Autodesk Inventor part; units mm, degrees
note: some values were not read from the file. Chosen so that the rebuilt part matches the saved one: direction of "Hole2".
(part 8 of 18)
  ellipse E33 centre (-86.9882, -23.0551) end of major axis (-85.4887, -23.0929) minor radius 0.2511 (-85.5525, -23.1627) -> (-87.7819, -22.8225) ccw
  ellipse E34 centre (-87.3359, -36.8531) end of major axis (-88.1356, -36.833) minor radius 0.1339 (-87.4465, -36.7177) -> (-87.4665, -36.7178) ccw
  ellipse E35 centre (-87.3607, -37.8387) end of major axis (-87.8606, -37.8261) minor radius 0.0837 (-87.1122, -37.9174) -> (-87.0891, -37.9156) ccw
  ellipse E36 centre (-87.3607, -37.8387) end of major axis (-86.8609, -37.8513) minor radius 0.0837 (-87.0358, -37.783) -> (-87.287, -37.7577) ccw
  line L78 (-105.3004, -36.9196) -> (-105.1861, -36.9462)
  ellipse E37 centre (-105.7695, -36.9513) end of major axis (-106.5469, -36.7626) minor radius 0.1369 (-105.4577, -36.8957) -> (-105.4762, -36.8899) ccw
  ellipse E38 centre (-106.002, -37.9088) end of major axis (-105.5161, -38.0267) minor radius 0.0856 (-105.735, -38.0451) -> (-105.8816, -37.8518) ccw
  ellipse E39 centre (-103.1271, -36.0379) end of major axis (-103.8852, -35.7824) minor radius 0.0023 (-103.715, -35.8383) -> (-103.8852, -35.7824) ccw
  line L79 (-101.9076, -36.989) -> (-102.0626, -37.449)
  line L80 (-103.888, -35.7905) -> (-103.8852, -35.7824)
  line L81 (-101.0026, -34.3039) -> (-99.7688, -30.6433)
  line L82 (-101.8233, -37.3232) -> (-102.0626, -37.449)
  line L83 (-102.0626, -37.449) -> (-102.0859, -37.4413)
  line L84 (-102.3857, -37.3402) -> (-102.0626, -37.449)
  line L85 (-90.6472, -35.9583) -> (-90.4914, -35.9237)
  ellipse E40 centre (-90.4117, -35.9087) end of major axis (-89.6305, -35.736) minor radius 0.0026 (-90.363, -35.8954) -> (-90.4914, -35.9237) ccw
  ellipse E41 centre (-90.4117, -35.9087) end of major axis (-89.6305, -35.736) minor radius 0.0026 (-90.2467, -35.8697) -> (-90.36, -35.8947) ccw
  ellipse E42 centre (-90.4117, -35.9087) end of major axis (-89.6305, -35.736) minor radius 0.0026 (-89.6305, -35.736) -> (-90.0478, -35.8259) ccw
  line L86 (-89.6301, -35.738) -> (-89.6305, -35.736)
  ellipse E43 centre (-87.6822, -37.9556) end of major axis (-86.8871, -37.8673) minor radius 0.2631 (-88.3686, -38.1574) -> (-88.2224, -38.2033) ccw
  ellipse E44 centre (-87.6822, -37.9556) end of major axis (-86.8871, -37.8673) minor radius 0.2631 (-87.1208, -38.0875) -> (-86.9563, -37.9921) ccw
  ellipse E45 centre (-106.3209, -37.9556) end of major axis (-107.116, -37.8673) minor radius 0.2631 (-106.8502, -37.7057) -> (-107.0012, -37.7511) ccw
  ellipse E46 centre (-106.3209, -37.9556) end of major axis (-107.116, -37.8673) minor radius 0.2631 (-107.0315, -37.7663) -> (-107.0404, -37.7715) ccw
  ellipse E47 centre (-106.3209, -37.9556) end of major axis (-107.116, -37.8673) minor radius 0.2631 (-107.107, -37.9186) -> (-106.8822, -38.0875) ccw
  ellipse E48 centre (-106.3209, -37.9556) end of major axis (-105.5258, -38.044) minor radius 0.2631 (-105.7807, -38.2033) -> (-105.6345, -38.1574) ccw
  line L87 (-92.5959, -36.6984) -> (-92.477, -36.6522)
  ellipse E49 centre (-91.0664, -36.1069) end of major axis (-90.3205, -35.8175) minor radius 0.0025 (-90.9446, -36.0571) -> (-90.9611, -36.0635) ccw
  ellipse E50 centre (-91.0664, -36.1069) end of major axis (-90.3205, -35.8175) minor radius 0.0025 (-90.8503, -36.0205) -> (-90.8987, -36.0393) ccw
  ellipse E51 centre (-91.0664, -36.1069) end of major axis (-90.3205, -35.8175) minor radius 0.0025 (-90.3205, -35.8175) -> (-90.3921, -35.8441) ccw
  line L88 (-92.2341, -37.6306) -> (-92.5959, -36.6984)
  ellipse E52 centre (-90.3428, -37.9714) end of major axis (-91.0886, -38.2609) minor radius 0.0025 (-90.6436, -38.0858) -> (-90.6333, -38.0866) ccw
  line L89 (-91.0886, -38.2609) -> (-91.4504, -37.3286)
  line L90 (-90.3147, -35.8327) -> (-90.3205, -35.8175)
  line L91 (-92.5959, -36.6984) -> (-94.5282, -31.7193)
  line L92 (-91.4495, -37.3309) -> (-92.2341, -37.6306)
  line L93 (-92.2341, -37.6306) -> (-92.5845, -37.4453)
  ellipse E53 centre (-92.2567, -37.3201) end of major axis (-93.1315, -36.9354) minor radius 0.2554 (-93.1284, -37.0086) -> (-92.5845, -37.4453) ccw
  line L94 (-93.1284, -37.0086) -> (-94.6292, -33.1414)
  ellipse E54 centre (-90.7046, -37.0392) end of major axis (-91.4504, -37.3286) minor radius 0.0025 (-91.304, -37.2702) -> (-91.4504, -37.3286) ccw
  line L95 (-92.2341, -37.6306) -> (-91.3087, -37.2712)
  ellipse E55 centre (-90.3428, -37.9714) end of major axis (-90.8089, -38.1523) minor radius 0.0015 (-90.6412, -38.086) -> (-90.6357, -38.0864) ccw
  ellipse E56 centre (-88.3729, -36.9958) end of major axis (-89.1416, -37.2174) minor radius 0.1461 (-88.5826, -36.9079) -> (-88.8145, -36.9941) ccw
  line L96 (-88.8154, -36.977) -> (-88.5903, -36.9086)
  ellipse E57 centre (-88.1005, -37.9405) end of major axis (-88.5809, -38.079) minor radius 0.0913 (-88.1238, -37.8521) -> (-88.2596, -38.0743) ccw
  ellipse E58 centre (-88.1005, -37.9405) end of major axis (-88.8692, -38.1621) minor radius 0.1461 (-88.4277, -37.8939) -> (-88.3686, -38.1574) ccw
  line L97 (-88.8692, -38.1621) -> (-88.9803, -37.7768)
  line L98 (-96.3959, -34.9516) -> (-96.4243, -34.4948)
  line L99 (-101.4811, -37.3766) -> (-101.4038, -37.5126)
  line L100 (-101.4038, -37.5126) -> (-100.927, -37.4058)
  ellipse E59 centre (-99.6492, -37.9242) end of major axis (-100.4225, -38.1293) minor radius 0.1421 (-100.4225, -38.1293) -> (-100.0049, -38.1458) ccw
  line L101 (-100.4225, -38.1293) -> (-100.5976, -37.4691)
  line L102 (-106.2018, -35.7078) -> (-106.2106, -35.5345)
  line L103 (-105.4545, -35.6102) -> (-105.4515, -35.6707)
  ellipse E60 centre (-106.8036, -35.8807) end of major axis (-107.6025, -35.9211) minor radius 0.143 (-107.0863, -35.7606) -> (-107.6025, -35.9211) ccw
  line L104 (-106.806, -35.7377) -> (-105.2331, -35.6598)
  line L105 (-105.2331, -35.6598) -> (-105.2316, -35.6894)
  ellipse E61 centre (-106.7042, -37.846) end of major axis (-107.5032, -37.8864) minor radius 0.143 (-107.024, -37.7305) -> (-107.0468, -37.9921) ccw
  ellipse E62 centre (-106.7042, -37.846) end of major axis (-107.5032, -37.8864) minor radius 0.143 (-106.4334, -37.6981) -> (-106.7066, -37.703) ccw
  line L106 (-107.5032, -37.8864) -> (-107.6025, -35.9211)
  line L107 (-105.2331, -35.6598) -> (-105.2348, -35.6248)
  line L108 (-105.2865, -34.6021) -> (-105.328, -33.7811)
  line L109 (-106.4202, -35.7186) -> (-106.4309, -35.508)
  ellipse E63 centre (-107.4941, -22.222) end of major axis (-109.5814, -22.3275) minor radius 0.3735 (-108.146, -21.8986) -> (-109.5814, -22.3275) ccw
  ellipse E64 centre (-107.4494, -23.1063) end of major axis (-109.5367, -23.2119) minor radius 0.3735 (-108.1131, -22.7842) -> (-109.0841, -23.4189) ccw
  line L110 (-109.5814, -22.3275) -> (-109.5367, -23.2119)
  ellipse E65 centre (-107.4494, -23.1063) end of major axis (-108.9475, -23.1821) minor radius 0.2681 (-106.2292, -22.8909) -> (-108.7917, -23.2912) ccw
  ellipse E66 centre (-106.7042, -37.846) end of major axis (-107.2036, -37.8712) minor radius 0.0894 (-106.7198, -37.7573) -> (-106.8898, -37.9381) ccw
  line L111 (-103.5666, -35.7887) -> (-103.544, -35.3586)
  line L112 (-102.9282, -34.2217) -> (-102.9384, -34.416)
  line L113 (-102.9917, -35.4294) -> (-103.0151, -35.8748)
  ellipse E67 centre (-104.3252, -35.809) end of major axis (-105.1241, -35.767) minor radius 0.0026 (-104.4162, -35.8017) -> (-105.1241, -35.767) ccw
  line L114 (-104.4162, -35.8017) -> (-102.8537, -35.8832)
  line L115 (-102.8537, -35.8832) -> (-102.8551, -35.9105)
  ellipse E68 centre (-104.4302, -37.8062) end of major axis (-105.2291, -37.7643) minor radius 0.0026 (-104.7673, -37.7862) -> (-104.7579, -37.7914) ccw
  line L116 (-105.2291, -37.7643) -> (-105.1241, -35.767)
  line L117 (-102.8537, -35.8832) -> (-102.7674, -34.2418)
  line L118 (-103.7279, -35.7784) -> (-103.7155, -35.5431)
  ellipse E69 centre (-104.4302, -37.8062) end of major axis (-104.9295, -37.78) minor radius 0.0016 (-104.7651, -37.7874) -> (-104.7602, -37.7901) ccw
  line L119 (-91.8056, -35.8014) -> (-92.3575, -33.1978)
  ellipse E70 centre (-90.3624, -35.9507) end of major axis (-88.9928, -35.6604) minor radius 0.2113 (-90.91, -35.8661) -> (-90.9339, -35.8727) ccw
  line L120 (-90.9872, -35.5021) -> (-90.91, -35.8661)
  line L121 (-91.9378, -36.3888) -> (-91.8413, -36.3397)
  line L122 (-90.91, -35.8661) -> (-90.8335, -35.8271)
  line L123 (-91.9378, -36.3888) -> (-90.398, -36.0813)
  ellipse E71 centre (-90.3624, -35.9507) end of major axis (-89.5798, -35.7848) minor radius 0.1207 (-90.398, -36.0813) -> (-89.7408, -35.747) ccw
  line L124 (-89.7408, -35.747) -> (-90.657, -35.7482)
  line L125 (-91.7329, -37.3559) -> (-91.9378, -36.3888)
  ellipse E72 centre (-89.9524, -37.8848) end of major axis (-90.7351, -38.0507) minor radius 0.1207 (-90.6436, -38.0858) -> (-89.2358, -37.7862) ccw
  line L126 (-89.5781, -35.7926) -> (-89.5798, -35.7848)
  line L127 (-91.9378, -36.3888) -> (-92.609, -33.2223)
  line L128 (-91.7329, -37.3559) -> (-92.0546, -37.0982)
  ellipse E73 centre (-91.7375, -36.9369) end of major axis (-92.5311, -36.3716) minor radius 0.32 (-92.5473, -36.4923) -> (-92.0546, -37.0982) ccw
  line L129 (-92.5473, -36.4923) -> (-93.8742, -30.2315)
  line L130 (-91.7329, -37.3559) -> (-90.193, -37.0483)
  line L131 (-89.3251, -35.7753) -> (-89.3885, -35.2136)
  line L132 (-88.4512, -35.6057) -> (-88.4408, -35.6984)
  line L133 (-88.8708, -35.9234) -> (-88.0017, -35.8236)
  ellipse E74 centre (-87.9255, -35.8321) end of major axis (-87.1305, -35.7424) minor radius 0.017 (-87.1432, -35.7409) -> (-88.0017, -35.8236) ccw
  ellipse E75 centre (-87.7014, -37.819) end of major axis (-88.4963, -37.9087) minor radius 0.017 (-86.9791, -37.7305) -> (-88.4277, -37.8939) ccw
  line L134 (-89.5896, -35.7345) -> (-89.6468, -35.2274)
  ellipse E76 centre (-89.4829, -22.0228) end of major axis (-87.406, -21.7886) minor radius 0.0445 (-87.4742, -21.785) -> (-87.8996, -21.8153) ccw
  ellipse E77 centre (-89.382, -22.9169) end of major axis (-87.3052, -22.6827) minor radius 0.0445 (-87.376, -22.6792) -> (-87.7951, -22.7091) ccw
  ellipse E78 centre (-87.8134, -36.8256) end of major axis (-88.6084, -36.9152) minor radius 0.017 (-87.8896, -36.8171) -> (-88.5826, -36.9079) ccw
  line L135 (-88.8182, -36.9237) -> (-87.8896, -36.8171)
  ellipse E79 centre (-87.7014, -37.819) end of major axis (-88.1982, -37.8751) minor radius 0.0106 (-87.2268, -37.7624) -> (-88.1906, -37.8723) ccw
  line L136 (-95.4221, -34.9516) -> (-95.3724, -34.4948)
  line L137 (-93.3346, -36.8473) -> (-94.4853, -36.841)
  line L138 (-94.3267, -37.4213) -> (-93.0147, -37.4285)
  line L139 (-93.0147, -37.4285) -> (-92.9086, -37.2552)
  ellipse E80 centre (-93.5822, -37.2515) end of major axis (-92.8706, -37.0672) minor radius 0.3717 (-93.1865, -36.8589) -> (-93.3346, -36.8473) ccw
  ellipse E81 centre (-93.5822, -37.2515) end of major axis (-92.8706, -37.0672) minor radius 0.3717 (-92.9086, -37.2552) -> (-92.9039, -37.2474) ccw
  ellipse E82 centre (-94.7288, -37.9666) end of major axis (-93.9335, -38.0531) minor radius 0.2736 (-94.1139, -38.2002) -> (-93.9982, -38.1458) ccw
  line L140 (-98.4172, -34.9516) -> (-98.4669, -34.4948)
  ellipse E83 centre (-100.2771, -37.2761) end of major axis (-99.5693, -37.3693) minor radius 0.4004 (-100.4443, -36.8697) -> (-100.9668, -37.3091) ccw
  line L141 (-100.9854, -37.2376) -> (-101.0007, -37.0971)
  line L142 (-99.5135, -36.8252) -> (-100.4443, -36.8697)
  line L143 (-100.9668, -37.3091) -> (-100.8951, -37.4833)
  line L144 (-100.8951, -37.4833) -> (-99.6774, -37.4251)
  ellipse E84 centre (-99.2743, -37.9666) end of major axis (-100.0696, -38.0531) minor radius 0.2736 (-100.0049, -38.1458) -> (-99.8891, -38.2002) ccw
  ellipse E85 centre (-106.0776, -35.8321) end of major axis (-106.8726, -35.7424) minor radius 0.017 (-106.0833, -35.8143) -> (-106.8599, -35.7409) ccw
  line L145 (-106.0833, -35.8143) -> (-105.1322, -35.9214)
  ellipse E86 centre (-106.3017, -37.819) end of major axis (-107.0967, -37.7294) minor radius 0.017 (-105.5754, -37.8939) -> (-107.024, -37.7305) ccw
  line L146 (-104.4898, -35.7366) -> (-104.4319, -35.2234)
  ellipse E87 centre (-104.5202, -22.0228) end of major axis (-106.5971, -21.7886) minor radius 0.0445 (-106.1035, -21.8153) -> (-106.5971, -21.7886) ccw
  ellipse E88 centre (-104.6211, -22.9169) end of major axis (-106.6979, -22.6827) minor radius 0.0445 (-106.208, -22.7091) -> (-106.627, -22.6792) ccw
  line L147 (-106.1954, -36.8078) -> (-105.1848, -36.9215)
  ellipse E89 centre (-106.1897, -36.8256) end of major axis (-105.3947, -36.9152) minor radius 0.017 (-105.4205, -36.9079) -> (-106.1954, -36.8078) ccw
  ellipse E90 centre (-106.3017, -37.819) end of major axis (-106.7986, -37.763) minor radius 0.0106 (-105.8581, -37.8739) -> (-106.7505, -37.773) ccw
  line L148 (-103.1826, -35.8132) -> (-104.1672, -35.7504)
  ellipse E91 centre (-103.6407, -35.9507) end of major axis (-104.4233, -35.7848) minor radius 0.1207 (-104.1672, -35.7504) -> (-103.7453, -36.0513) ccw
  line L149 (-103.7453, -36.0513) -> (-102.2177, -36.3998)
  line L150 (-102.2177, -36.3998) -> (-102.4227, -37.3668)
  ellipse E92 centre (-104.0506, -37.8848) end of major axis (-104.8333, -37.7189) minor radius 0.1207 (-104.7673, -37.7862) -> (-103.3595, -38.0858) ccw
  line L151 (-104.425, -35.7926) -> (-104.4233, -35.7848)
  line L152 (-102.2505, -36.3764) -> (-102.2177, -36.3998)
  line L153 (-102.2177, -36.3998) -> (-101.5416, -33.2099)
  ellipse E93 centre (-102.2845, -36.9758) end of major axis (-101.4721, -36.4169) minor radius 0.2359 (-102.0808, -37.121) -> (-101.4724, -36.5094) ccw
  line L154 (-101.4046, -36.2006) -> (-100.1521, -30.2914)
  line L155 (-102.0808, -37.121) -> (-102.4227, -37.3668)
  line L156 (-103.9503, -37.0183) -> (-102.4227, -37.3668)
  line L157 (-91.0541, -35.879) -> (-91.0769, -35.4447)
  line L158 (-90.2308, -35.4655) -> (-90.216, -35.7476)
  line L159 (-91.2994, -35.892) -> (-89.73, -35.8092)
  ellipse E94 centre (-89.6779, -35.809) end of major axis (-88.879, -35.767) minor radius 0.0026 (-88.879, -35.767) -> (-89.73, -35.8092) ccw
  line L160 (-91.2968, -35.9413) -> (-91.2994, -35.892)
  ellipse E95 centre (-89.5729, -37.8062) end of major axis (-88.774, -37.7643) minor radius 0.0026 (-89.2452, -37.7914) -> (-89.2358, -37.7862) ccw
  line L161 (-88.774, -37.7643) -> (-88.879, -35.767)
  line L162 (-89.9702, -35.7439) -> (-89.9858, -35.4481)
  line L163 (-91.2994, -35.892) -> (-91.3855, -34.2529)
  ellipse E96 centre (-89.5729, -37.8062) end of major axis (-89.0736, -37.78) minor radius 0.0016 (-89.2428, -37.7901) -> (-89.238, -37.7874) ccw
  line L164 (-88.5794, -35.6942) -> (-88.5755, -35.6163)
  line L165 (-87.6584, -35.5185) -> (-87.6687, -35.7223)
  line L166 (-88.8445, -35.686) -> (-87.2794, -35.7344)
  ellipse E97 centre (-87.1995, -35.8807) end of major axis (-86.4005, -35.9211) minor radius 0.143 (-86.4005, -35.9211) -> (-86.9168, -35.7606) ccw
  line L167 (-88.8467, -35.7306) -> (-88.8445, -35.686)
  ellipse E98 centre (-87.2989, -37.846) end of major axis (-86.4999, -37.8864) minor radius 0.143 (-86.639, -37.959) -> (-86.9791, -37.7305) ccw
  line L168 (-86.4999, -37.8864) -> (-86.4005, -35.9211)
  line L169 (-87.4036, -35.7305) -> (-87.3912, -35.485)
  line L170 (-88.8445, -35.686) -> (-88.8346, -35.4897)
  line L171 (-88.7547, -33.9096) -> (-88.742, -33.6588)
  ellipse E99 centre (-86.509, -22.222) end of major axis (-84.4216, -22.3275) minor radius 0.3735 (-84.4216, -22.3275) -> (-85.857, -21.8986) ccw
  ellipse E100 centre (-86.5537, -23.1063) end of major axis (-84.4663, -23.2119) minor radius 0.3735 (-84.8558, -23.407) -> (-85.89, -22.7842) ccw
  line L172 (-84.4216, -22.3275) -> (-84.4663, -23.2119)
  ellipse E101 centre (-86.5537, -23.1063) end of major axis (-85.0556, -23.1821) minor radius 0.2681 (-85.1981, -23.287) -> (-87.7739, -22.8909) ccw
  ellipse E102 centre (-87.2989, -37.846) end of major axis (-86.7995, -37.8712) minor radius 0.0894 (-87.1133, -37.9381) -> (-87.2833, -37.7573) ccw
  line L173 (-92.9989, -37.4027) -> (-92.5139, -37.5)
  line L174 (-92.5139, -37.5) -> (-92.5046, -37.4875)
  ellipse E103 centre (-94.3538, -37.9242) end of major axis (-93.5806, -38.1293) minor radius 0.1421 (-93.9982, -38.1458) -> (-93.5806, -38.1293) ccw
  line L175 (-93.5806, -38.1293) -> (-93.3941, -37.4264)
  line L176 (-97.4502, -34.9516) -> (-97.4218, -34.4948)
  line L177 (-105.396, -36.9102) -> (-105.1873, -36.9692)
  ellipse E104 centre (-105.6302, -36.9958) end of major axis (-106.3989, -36.7741) minor radius 0.1461 (-105.1886, -36.9941) -> (-105.4205, -36.9079) ccw
  ellipse E105 centre (-105.9026, -37.9405) end of major axis (-105.4222, -38.079) minor radius 0.0913 (-105.7434, -38.0743) -> (-105.8793, -37.8521) ccw
  ellipse E106 centre (-105.9026, -37.9405) end of major axis (-105.1339, -38.1621) minor radius 0.1461 (-105.6345, -38.1574) -> (-105.5754, -37.8939) ccw
  line L178 (-105.1339, -38.1621) -> (-105.0228, -37.7768)
  ellipse E107 centre (-102.9367, -36.1069) end of major axis (-103.6825, -35.8175) minor radius 0.0025 (-103.6284, -35.8375) -> (-103.6825, -35.8175) ccw
  ellipse E108 centre (-102.9367, -36.1069) end of major axis (-102.1909, -36.3963) minor radius 0.0025 (-103.6123, -35.8436) -> (-103.6145, -35.8428) ccw
  line L179 (-101.5514, -36.6414) -> (-101.5406, -36.6456)
  line L180 (-101.5406, -36.6456) -> (-101.9024, -37.5779)
  ellipse E109 centre (-103.6603, -37.9714) end of major axis (-102.9145, -38.2609) minor radius 0.0025 (-103.3698, -38.0866) -> (-103.3595, -38.0858) ccw
  line L181 (-103.6862, -35.8269) -> (-103.6825, -35.8175)
  line L182 (-102.9145, -38.2609) -> (-102.5558, -37.3365)
  line L183 (-101.5406, -36.6456) -> (-101.5249, -36.6051)
  line L184 (-101.4524, -36.4183) -> (-99.5384, -31.4865)
  ellipse E110 centre (-101.7527, -37.3167) end of major axis (-100.8603, -36.9239) minor radius 0.1687 (-101.5309, -37.4006) -> (-100.8618, -36.956) ccw
  line L185 (-100.8618, -36.956) -> (-99.2082, -32.6952)
  line L186 (-101.5309, -37.4006) -> (-101.9024, -37.5779)
  line L187 (-101.9024, -37.5779) -> (-102.5174, -37.3453)
  line L188 (-102.4809, -37.3536) -> (-101.9024, -37.5779)
  ellipse E111 centre (-103.6603, -37.9714) end of major axis (-103.1942, -38.1523) minor radius 0.0015 (-103.3673, -38.0864) -> (-103.3619, -38.086) ccw
  line L189 (-91.6135, -36.1343) -> (-90.3354, -35.89)
  ellipse E112 centre (-90.2843, -35.8825) end of major axis (-89.4985, -35.7324) minor radius 0.0022 (-90.1356, -35.8519) -> (-90.3354, -35.89) ccw
  ellipse E113 centre (-90.2843, -35.8825) end of major axis (-89.4985, -35.7324) minor radius 0.0022 (-89.4985, -35.7324) -> (-89.9806, -35.8224) ccw
  line L190 (-89.4972, -35.7389) -> (-89.4985, -35.7324)
  line L191 (-88.8738, -35.8662) -> (-87.9337, -35.7613)
  ellipse E114 centre (-89.105, -23.1133) end of major axis (-87.6121, -22.9671) minor radius 0.2416 (-87.6775, -22.906) -> (-87.7756, -22.876) ccw
  ellipse E115 centre (-89.105, -23.1133) end of major axis (-87.0249, -22.9096) minor radius 0.3366 (-87.0984, -22.8327) -> (-87.1043, -22.8298) ccw
  ellipse E116 centre (-87.662, -37.847) end of major axis (-88.1596, -37.8957) minor radius 0.0805 (-88.0954, -37.8486) -> (-88.1457, -37.8741) ccw
  ellipse E117 centre (-87.662, -37.847) end of major axis (-87.1643, -37.7982) minor radius 0.0805 (-87.1746, -37.7841) -> (-87.2888, -37.7579) ccw
  ellipse E118 centre (-103.7126, -35.9107) end of major axis (-102.9272, -36.0627) minor radius 0.0868 (-103.7664, -35.8122) -> (-104.3602, -35.7368) ccw
  line L192 (-103.7664, -35.8122) -> (-103.5882, -35.8449)
  line L193 (-91.0063, -36.0712) -> (-90.7647, -35.9995)
  ellipse E119 centre (-90.7187, -35.9881) end of major axis (-89.9517, -35.7606) minor radius 0.0022 (-90.572, -35.9424) -> (-90.7647, -35.9995) ccw
  ellipse E120 centre (-90.7187, -35.9881) end of major axis (-89.9517, -35.7606) minor radius 0.0022 (-90.5008, -35.9213) -> (-90.5033, -35.9221) ccw
  ellipse E121 centre (-90.7187, -35.9881) end of major axis (-89.9517, -35.7606) minor radius 0.0022 (-89.9522, -35.7607) -> (-90.2056, -35.8343) ccw
  line L194 (-91.9875, -37.4055) -> (-92.0863, -37.0725)
  line L195 (-94.0142, -29.8718) -> (-94.0243, -29.8748)
  line L196 (-93.2708, -33.0786) -> (-94.1186, -30.2201)
  line L197 (-91.9762, -37.4022) -> (-91.9875, -37.4055)
  line L198 (-91.9875, -37.4055) -> (-92.0512, -37.3656)
  line L199 (-91.9875, -37.4055) -> (-91.7565, -37.3369)
  line L200 (-88.4153, -35.8419) -> (-88.3977, -35.8381)
  ellipse E122 centre (-88.3231, -35.9536) end of major axis (-87.5398, -35.791) minor radius 0.1285 (-88.162, -35.7927) -> (-88.3977, -35.8381) ccw
  line L201 (-88.8173, -36.9397) -> (-88.7541, -36.9259)
  ellipse E123 centre (-87.9219, -37.8864) end of major axis (-88.4114, -37.9881) minor radius 0.0803 (-88.1213, -37.8518) -> (-88.2768, -38.0146) ccw
  ellipse E124 centre (-106.6098, -35.8587) end of major axis (-107.4098, -35.864) minor radius 0.1258 (-106.5896, -35.7328) -> (-107.4098, -35.864) ccw
  line L202 (-106.5896, -35.7328) -> (-105.8749, -35.7311)
  line L203 (-105.0369, -35.729) -> (-105.0153, -35.729)
  line L204 (-105.0153, -35.729) -> (-105.0151, -35.7582)
  ellipse E125 centre (-106.5968, -37.8338) end of major axis (-107.3967, -37.8391) minor radius 0.1258 (-106.3119, -37.7144) -> (-106.5766, -37.7079) ccw
  line L205 (-105.0153, -35.729) -> (-105.0188, -35.1913)
  line L206 (-105.0254, -34.1869) -> (-105.0288, -33.6714)
  ellipse E126 centre (-106.7002, -22.132) end of major axis (-108.7902, -22.1457) minor radius 0.3286 (-106.8625, -21.8053) -> (-107.8913, -21.8696) ccw
  ellipse E127 centre (-106.6944, -23.0207) end of major axis (-108.7843, -23.0345) minor radius 0.3286 (-106.939, -22.6959) -> (-107.8776, -22.7574) ccw
  ellipse E128 centre (-106.6944, -23.0207) end of major axis (-108.1943, -23.0306) minor radius 0.2359 (-106.2179, -22.794) -> (-108.192, -23.0435) ccw
  ellipse E129 centre (-106.5968, -37.8338) end of major axis (-107.0967, -37.8371) minor radius 0.0786 (-106.7124, -37.7581) -> (-106.8918, -37.8992) ccw
  ellipse E130 centre (-104.1835, -35.8187) end of major axis (-104.9807, -35.7515) minor radius 0.0022 (-104.2673, -35.8094) -> (-104.9807, -35.7515) ccw
  line L207 (-104.9814, -35.7603) -> (-104.9807, -35.7515)
  line L208 (-91.6125, -36.1341) -> (-92.1617, -33.1749)
  line L209 (-91.8337, -36.2617) -> (-91.608, -36.1759)
  line L210 (-91.8337, -36.2617) -> (-90.286, -35.9829)
  ellipse E131 centre (-90.2575, -35.8989) end of major axis (-89.4709, -35.7529) minor radius 0.0775 (-90.286, -35.9829) -> (-89.6305, -35.7361) ccw
  ellipse E132 centre (-90.2575, -35.8989) end of major axis (-91.044, -36.0449) minor radius 0.0775 (-89.6322, -35.7362) -> (-89.6374, -35.7365) ccw
  line L211 (-89.6374, -35.7365) -> (-89.6817, -35.7389)
  line L212 (-91.8274, -36.2956) -> (-91.8337, -36.2617)
  line L213 (-89.4646, -35.7868) -> (-89.4709, -35.7529)
  line L214 (-91.8337, -36.2617) -> (-92.0935, -34.8619)
  line L215 (-89.2509, -35.7692) -> (-89.3057, -35.2091)
  line L216 (-88.8726, -35.8885) -> (-87.9213, -35.7915)
  ellipse E133 centre (-87.8582, -35.8315) end of major axis (-87.062, -35.7537) minor radius 0.046 (-87.12, -35.7423) -> (-87.9213, -35.7915) ccw
  line L217 (-89.505, -35.7334) -> (-89.5549, -35.2225)
  ellipse E134 centre (-89.2075, -22.0202) end of major axis (-87.1274, -21.817) minor radius 0.1201 (-87.1406, -21.8053) -> (-87.9015, -21.7991) ccw
  ellipse E135 centre (-89.1201, -22.9144) end of major axis (-87.04, -22.7112) minor radius 0.1201 (-87.0641, -22.6959) -> (-87.3086, -22.6787) ccw
  ellipse E136 centre (-89.1201, -22.9144) end of major axis (-87.6272, -22.7686) minor radius 0.0862 (-87.7819, -22.8225) -> (-87.7909, -22.7456) ccw
  ellipse E137 centre (-87.6641, -37.8187) end of major axis (-87.1665, -37.7701) minor radius 0.0287 (-87.2077, -37.7627) -> (-87.2241, -37.7624) ccw
  line L218 (-104.7135, -35.2082) -> (-104.7682, -35.7679)
  ellipse E138 centre (-106.1448, -35.8315) end of major axis (-106.9411, -35.7537) minor radius 0.046 (-106.1282, -35.7869) -> (-106.8831, -35.7423) ccw
  line L219 (-106.1282, -35.7869) -> (-105.1303, -35.8853)
  ellipse E139 centre (-104.7956, -22.0202) end of major axis (-106.8757, -21.817) minor radius 0.1201 (-106.1016, -21.7991) -> (-106.8625, -21.8053) ccw
  ellipse E140 centre (-104.883, -22.9144) end of major axis (-106.9631, -22.7112) minor radius 0.1201 (-106.6944, -22.6787) -> (-106.939, -22.6959) ccw
  ellipse E141 centre (-104.883, -22.9144) end of major axis (-106.3759, -22.7686) minor radius 0.0862 (-106.2122, -22.7456) -> (-106.2212, -22.8225) ccw
  ellipse E142 centre (-106.339, -37.8187) end of major axis (-105.8413, -37.8673) minor radius 0.0287 (-105.8603, -37.8732) -> (-105.8816, -37.8518) ccw
  ellipse E143 centre (-106.339, -37.8187) end of major axis (-106.8366, -37.7701) minor radius 0.0287 (-106.6189, -37.7676) -> (-106.8132, -37.7813) ccw
  line L220 (-101.8881, -33.1694) -> (-102.4323, -36.102)
  ellipse E144 centre (-103.7456, -35.8989) end of major axis (-104.5322, -35.7529) minor radius 0.0775 (-104.3602, -35.7368) -> (-103.8216, -35.9634) ccw
  line L221 (-103.8216, -35.9634) -> (-102.3431, -36.2495)
  line L222 (-104.5385, -35.7868) -> (-104.5322, -35.7529)
  line L223 (-91.4265, -35.9522) -> (-89.8591, -35.8198)
  ellipse E145 centre (-89.8196, -35.8187) end of major axis (-89.0224, -35.7515) minor radius 0.0022 (-89.7375, -35.8096) -> (-89.8591, -35.8198) ccw
  ellipse E146 centre (-89.8196, -35.8187) end of major axis (-89.0224, -35.7515) minor radius 0.0022 (-89.0224, -35.7515) -> (-89.7373, -35.8096) ccw
  line L224 (-91.4143, -36.0962) -> (-91.4265, -35.9522)
  line L225 (-89.0217, -35.7603) -> (-89.0224, -35.7515)
  line L226 (-91.4265, -35.9522) -> (-91.5707, -34.2426)
  line L227 (-91.6631, -33.1465) -> (-91.6656, -33.1169)
  line L228 (-87.9002, -35.5469) -> (-87.9013, -35.7151)
  line L229 (-89.0294, -35.7435) -> (-87.46, -35.7329)
  ellipse E147 centre (-87.3933, -35.8587) end of major axis (-86.5933, -35.864) minor radius 0.1258 (-86.9598, -35.7558) -> (-87.46, -35.7329) ccw
  line L230 (-89.0294, -35.7518) -> (-89.0294, -35.7435)
  line L231 (-89.0294, -35.7435) -> (-89.0258, -35.1936)
  line L232 (-89.0191, -34.1888) -> (-89.0139, -33.3998)
  ellipse E148 centre (-87.3029, -22.132) end of major axis (-89.3928, -22.1182) minor radius 0.3286 (-86.1118, -21.8696) -> (-87.1406, -21.8053) ccw
  ellipse E149 centre (-87.3087, -23.0207) end of major axis (-89.3987, -23.007) minor radius 0.3286 (-86.1255, -22.7574) -> (-87.0641, -22.6959) ccw
  ellipse E150 centre (-87.3087, -23.0207) end of major axis (-85.8087, -23.0306) minor radius 0.2359 (-85.8267, -23.0666) -> (-87.7852, -22.794) ccw
  ellipse E151 centre (-87.3998, -36.8463) end of major axis (-88.1998, -36.841) minor radius 0.1258 (-87.4666, -36.7205) -> (-87.7879, -36.7338) ccw
  ellipse E152 centre (-87.4063, -37.8338) end of major axis (-86.9063, -37.8371) minor radius 0.0786 (-87.0538, -37.7803) -> (-87.2907, -37.7581) ccw
  line L233 (-105.197, -36.9311) -> (-105.1854, -36.9335)
  ellipse E153 centre (-106.0812, -37.8864) end of major axis (-105.5917, -37.9881) minor radius 0.0803 (-105.7262, -38.0146) -> (-105.8818, -37.8518) ccw
  ellipse E154 centre (-103.2844, -35.9881) end of major axis (-104.0514, -35.7606) minor radius 0.0022 (-103.7988, -35.8339) -> (-104.0508, -35.7607) ccw
  line L234 (-100.4876, -31.8742) -> (-99.9384, -30.0226)
  line L235 (-99.9791, -29.8737) -> (-99.9886, -29.871)
  ellipse E155 centre (-89.1052, -33.362) end of major axis (-88.2646, -33.1579) minor radius 0.1481 (-89.2261, -33.2398) -> (-89.2962, -33.2587) ccw
  ellipse E156 centre (-89.1052, -33.362) end of major axis (-88.2646, -33.1579) minor radius 0.1481 (-89.0355, -33.1939) -> (-89.0825, -33.2045) ccw
  ellipse E157 centre (-106.7756, -32.5501) end of major axis (-106.3188, -32.5386) minor radius 0.0765 (-106.3956, -32.4983) -> (-106.9486, -32.4835) ccw
  ellipse E158 centre (-106.7756, -32.5501) end of major axis (-107.6404, -32.5719) minor radius 0.1448 (-106.2741, -32.4198) -> (-107.4825, -32.6508) ccw
  ellipse E159 centre (-106.8005, -31.5645) end of major axis (-107.6652, -31.5863) minor radius 0.1448 (-106.5829, -31.419) -> (-107.6652, -31.5863) ccw
  line L236 (-107.6652, -31.5863) -> (-107.6404, -32.5719)
  ellipse E160 centre (-104.0594, -33.2898) end of major axis (-104.9222, -33.228) minor radius 0.0025 (-103.9619, -33.2942) -> (-104.7062, -33.2451) ccw
  line L237 (-104.8929, -32.8184) -> (-104.9222, -33.228)
  ellipse E161 centre (-88.1251, -33.5826) end of major axis (-88.9854, -33.6727) minor radius 0.037 (-87.2688, -33.4968) -> (-88.9661, -33.6784) ccw
  ellipse E162 centre (-88.2291, -32.589) end of major axis (-87.3688, -32.4989) minor radius 0.037 (-87.3688, -32.4989) -> (-88.6087, -32.5953) ccw
  line L238 (-87.3688, -32.4989) -> (-87.2648, -33.4926)
  line L239 (-89.0753, -32.8143) -> (-88.9854, -33.6727)
  ellipse E163 centre (-105.878, -33.5826) end of major axis (-106.7383, -33.4926) minor radius 0.037 (-105.0177, -33.6728) -> (-106.7342, -33.4968) ccw
  ellipse E164 centre (-105.774, -32.589) end of major axis (-106.6343, -32.4989) minor radius 0.037 (-105.3944, -32.5953) -> (-106.6343, -32.4989) ccw
  line L240 (-104.9278, -32.8143) -> (-105.0177, -33.6727)
  line L241 (-106.6343, -32.4989) -> (-106.7383, -33.4926)
  ellipse E165 centre (-89.9436, -33.2898) end of major axis (-89.0808, -33.228) minor radius 0.0025 (-89.2969, -33.2451) -> (-90.0412, -33.2942) ccw
  line L242 (-89.1102, -32.8184) -> (-89.0808, -33.228)
  ellipse E166 centre (-87.2275, -32.5501) end of major axis (-86.7706, -32.5616) minor radius 0.0765 (-87.0545, -32.4835) -> (-87.6075, -32.4983) ccw
  ellipse E167 centre (-87.2275, -32.5501) end of major axis (-86.3627, -32.5719) minor radius 0.1448 (-86.5206, -32.6508) -> (-87.729, -32.4198) ccw
  ellipse E168 centre (-87.2026, -31.5645) end of major axis (-86.3379, -31.5863) minor radius 0.1448 (-86.3379, -31.5863) -> (-87.4202, -31.419) ccw
  line L243 (-86.3379, -31.5863) -> (-86.3627, -32.5719)
  ellipse E169 centre (-90.5404, -35.3268) end of major axis (-90.9866, -35.4255) minor radius 0.0015 (-90.2127, -35.2533) -> (-90.975, -35.4233) ccw
  ellipse E170 centre (-90.5404, -35.3268) end of major axis (-89.6958, -35.14) minor radius 0.0028 (-90.1297, -35.2335) -> (-91.2208, -35.4756) ccw
  ellipse E171 centre (-90.7563, -34.3504) end of major axis (-89.9117, -34.1636) minor radius 0.0028 (-90.0298, -34.1883) -> (-91.3368, -34.4767) ccw
  line L244 (-87.227, -34.3409) -> (-87.2154, -34.4433)
  line L245 (-106.7761, -34.3409) -> (-106.7877, -34.4433)
  ellipse E172 centre (-103.4627, -35.3268) end of major axis (-103.0165, -35.4255) minor radius 0.0015 (-103.0281, -35.4233) -> (-103.7904, -35.2533) ccw
  ellipse E173 centre (-103.4627, -35.3268) end of major axis (-102.6181, -35.5136) minor radius 0.0028 (-102.9313, -35.4421) -> (-103.8733, -35.2335) ccw
  ellipse E174 centre (-103.2468, -34.3504) end of major axis (-102.4022, -34.5372) minor radius 0.0028 (-102.8483, -34.436) -> (-103.9733, -34.1883) ccw
  ellipse E175 centre (-90.5313, -35.4526) end of major axis (-90.0855, -35.3522) minor radius 0.0774 (-90.3319, -35.48) -> (-90.9345, -35.5066) ccw
  ellipse E176 centre (-90.5313, -35.4526) end of major axis (-89.6874, -35.2627) minor radius 0.1465 (-90.9893, -35.4264) -> (-91.0763, -35.4569) ccw
  ellipse E177 centre (-90.5313, -35.4526) end of major axis (-89.6874, -35.2627) minor radius 0.1465 (-90.0773, -35.48) -> (-89.7284, -35.2308) ccw
  line L246 (-89.6948, -35.2298) -> (-89.6874, -35.2627)
  ellipse E178 centre (-103.4717, -35.4526) end of major axis (-103.9176, -35.3522) minor radius 0.0774 (-103.063, -35.51) -> (-103.5846, -35.5047) ccw
  ellipse E179 centre (-103.4717, -35.4526) end of major axis (-102.6279, -35.6425) minor radius 0.1465 (-102.9919, -35.4338) -> (-103.0137, -35.4264) ccw
  ellipse E180 centre (-103.4717, -35.4526) end of major axis (-104.3156, -35.2627) minor radius 0.1465 (-104.2747, -35.2308) -> (-103.7152, -35.5432) ccw
  line L247 (-104.3082, -35.2298) -> (-104.3156, -35.2627)
  ellipse E181 centre (-91.7653, -34.3058) end of major axis (-90.9589, -33.9928) minor radius 0.0027 (-91.5915, -34.2356) -> (-91.9398, -34.3707) ccw
  ellipse E182 centre (-92.1271, -33.3735) end of major axis (-91.3207, -33.0606) minor radius 0.0027 (-91.8187, -33.2512) -> (-92.1255, -33.3701) ccw
  ellipse E183 centre (-89.1876, -34.1702) end of major axis (-88.3565, -33.9306) minor radius 0.158 (-89.0531, -33.9708) -> (-89.2559, -34.0255) ccw
  ellipse E184 centre (-89.1876, -34.1702) end of major axis (-88.3565, -33.9306) minor radius 0.158 (-88.662, -33.8968) -> (-88.9994, -33.958) ccw
  ellipse E185 centre (-106.8812, -34.3458) end of major axis (-107.3376, -34.3689) minor radius 0.0817 (-106.6537, -34.2638) -> (-106.7852, -34.4211) ccw
  ellipse E186 centre (-106.8812, -34.3458) end of major axis (-107.7451, -34.3895) minor radius 0.1546 (-106.411, -34.1929) -> (-106.7974, -34.4958) ccw
  ellipse E187 centre (-106.9308, -33.3632) end of major axis (-107.7947, -33.4069) minor radius 0.1546 (-106.708, -33.2027) -> (-107.7947, -33.4069) ccw
  line L248 (-107.7947, -33.4069) -> (-107.7451, -34.3895)
  ellipse E188 centre (-104.2947, -35.2278) end of major axis (-104.751, -35.2038) minor radius 0.0015 (-103.9002, -35.2493) -> (-104.0669, -35.2411) ccw
  ellipse E189 centre (-104.2947, -35.2278) end of major axis (-105.1585, -35.1824) minor radius 0.0028 (-103.7902, -35.2521) -> (-104.3083, -35.2299) ccw
  ellipse E190 centre (-104.2422, -34.2292) end of major axis (-103.3784, -34.2746) minor radius 0.0028 (-103.4994, -34.2668) -> (-103.6527, -34.2581) ccw
  ellipse E191 centre (-104.2422, -34.2292) end of major axis (-105.106, -34.1838) minor radius 0.0028 (-103.7401, -34.2533) -> (-105.106, -34.1838) ccw
  line L249 (-105.106, -34.1838) -> (-105.1585, -35.1824)
  ellipse E192 centre (-90.7686, -34.0339) end of major axis (-91.6148, -34.2133) minor radius 0.1305 (-91.6148, -34.2133) -> (-89.9224, -33.8546) ccw
  ellipse E193 centre (-90.9736, -33.0669) end of major axis (-91.8198, -33.2462) minor radius 0.1305 (-91.7075, -33.1522) -> (-90.1693, -32.9421) ccw
  line L250 (-90.1171, -32.936) -> (-89.9224, -33.8546)
  line L251 (-91.8198, -33.2462) -> (-91.6148, -34.2133)
  ellipse E194 centre (-87.959, -35.535) end of major axis (-87.5048, -35.4838) minor radius 0.0097
  ellipse E195 centre (-87.959, -35.535) end of major axis (-88.8185, -35.632) minor radius 0.0184 (-88.5755, -35.6175) -> (-88.803, -35.6337) ccw
  ellipse E196 centre (-88.071, -34.5416) end of major axis (-88.9306, -34.6385) minor radius 0.0184 (-87.2115, -34.4446) -> (-88.8739, -34.6254) ccw
  line L252 (-87.2115, -34.4446) -> (-87.0994, -35.4381)
  line L253 (-88.869, -35.1844) -> (-88.8185, -35.632)
  ellipse E197 centre (-106.0441, -35.535) end of major axis (-106.4982, -35.4838) minor radius 0.0097
  ellipse E198 centre (-106.0441, -35.535) end of major axis (-106.9037, -35.4381) minor radius 0.0184 (-105.1879, -35.6299) -> (-105.4543, -35.615) ccw
  ellipse E199 centre (-105.9321, -34.5416) end of major axis (-106.7916, -34.4446) minor radius 0.0184 (-105.1292, -34.6254) -> (-106.7916, -34.4446) ccw
  line L254 (-106.7916, -34.4446) -> (-106.9037, -35.4381)
  ellipse E200 centre (-103.2344, -34.0339) end of major axis (-104.0806, -33.8546) minor radius 0.1305 (-104.0806, -33.8546) -> (-102.3882, -34.2133) ccw
  ellipse E201 centre (-103.0295, -33.0669) end of major axis (-103.8757, -32.8875) minor radius 0.1305 (-103.8338, -32.9421) -> (-102.2144, -33.1994) ccw
  line L255 (-102.1833, -33.2462) -> (-102.3882, -34.2133)
  line L256 (-103.886, -32.936) -> (-104.0806, -33.8546)
  ellipse E202 centre (-89.7084, -35.2278) end of major axis (-90.1648, -35.2518) minor radius 0.0015 (-89.9362, -35.2411) -> (-90.1029, -35.2493) ccw
  ellipse E203 centre (-89.7084, -35.2278) end of major axis (-88.8446, -35.1824) minor radius 0.0028 (-89.6948, -35.2299) -> (-90.2129, -35.2521) ccw
  ellipse E204 centre (-89.7609, -34.2292) end of major axis (-88.8971, -34.1838) minor radius 0.0028 (-90.3504, -34.2581) -> (-90.5037, -34.2668) ccw
  ellipse E205 centre (-89.7609, -34.2292) end of major axis (-88.8971, -34.1838) minor radius 0.0028 (-88.8971, -34.1838) -> (-90.263, -34.2533) ccw
  line L257 (-88.8971, -34.1838) -> (-88.8446, -35.1824)
  ellipse E206 centre (-87.1219, -34.3458) end of major axis (-86.6655, -34.3689) minor radius 0.0817 (-87.2179, -34.4211) -> (-87.3494, -34.2638) ccw
  ellipse E207 centre (-87.1219, -34.3458) end of major axis (-86.258, -34.3895) minor radius 0.1546 (-87.2057, -34.4958) -> (-87.5921, -34.1929) ccw
  ellipse E208 centre (-87.0722, -33.3632) end of major axis (-86.2083, -33.4069) minor radius 0.1546 (-86.2083, -33.4069) -> (-87.2951, -33.2027) ccw
  line L258 (-86.2083, -33.4069) -> (-86.258, -34.3895)
  ellipse E209 centre (-104.8155, -34.1702) end of major axis (-103.9843, -34.4099) minor radius 0.158 (-104.7472, -34.0255) -> (-104.8217, -34.0043) ccw
  ellipse E210 centre (-102.2377, -34.3058) end of major axis (-101.4313, -34.6188) minor radius 0.0027 (-102.1078, -34.3534) -> (-102.2412, -34.3016) ccw
  ellipse E211 centre (-101.8759, -33.3735) end of major axis (-101.0695, -33.6865) minor radius 0.0027 (-101.9221, -33.3528) -> (-102.1106, -33.2798) ccw
  ellipse E212 centre (-88.4471, -29.6963) end of major axis (-87.5861, -29.6131) minor radius 0.2215 (-87.8663, -29.4796) -> (-87.9624, -29.4687) ccw
  ellipse E213 centre (-105.556, -29.6963) end of major axis (-104.695, -29.7796) minor radius 0.2215 (-106.0407, -29.4687) -> (-106.1368, -29.4796) ccw
  ellipse E214 centre (-106.6437, -30.7028) end of major axis (-106.1868, -30.6998) minor radius 0.0719 (-106.5062, -30.6334) -> (-106.8364, -30.6389) ccw
  ellipse E215 centre (-106.6437, -30.7028) end of major axis (-107.5087, -30.7085) minor radius 0.136 (-106.4997, -30.5678) -> (-107.5074, -30.7008) ccw
  ellipse E216 centre (-106.6503, -29.7153) end of major axis (-107.5152, -29.721) minor radius 0.136 (-106.0548, -29.6128) -> (-107.5103, -29.7063) ccw
  ellipse E217 centre (-88.2703, -31.6135) end of major axis (-87.8155, -31.5691) minor radius 0.0263 (-87.8178, -31.5722) -> (-87.8184, -31.5666) ccw
  ellipse E218 centre (-88.2703, -31.6135) end of major axis (-87.4094, -31.5294) minor radius 0.0497 (-87.4192, -31.5382) -> (-88.4553, -31.5828) ccw
  ellipse E219 centre (-88.3674, -30.6199) end of major axis (-87.5065, -30.5358) minor radius 0.0497 (-87.5065, -30.5358) -> (-88.3008, -30.5636) ccw
  line L259 (-87.5065, -30.5358) -> (-87.4094, -31.5294)
  ellipse E220 centre (-105.7328, -31.6135) end of major axis (-106.1876, -31.5691) minor radius 0.0263 (-106.1847, -31.5666) -> (-106.1853, -31.5722) ccw
  ellipse E221 centre (-105.7328, -31.6135) end of major axis (-106.5937, -31.5294) minor radius 0.0497 (-105.5478, -31.5828) -> (-106.5839, -31.5382) ccw
  ellipse E222 centre (-105.6357, -30.6199) end of major axis (-106.4966, -30.5358) minor radius 0.0497 (-105.7023, -30.5636) -> (-106.4966, -30.5358) ccw
  line L260 (-106.4966, -30.5358) -> (-106.5937, -31.5294)
  ellipse E223 centre (-87.3593, -30.7028) end of major axis (-86.9023, -30.7058) minor radius 0.0719 (-87.1667, -30.6389) -> (-87.4969, -30.6334) ccw
  ellipse E224 centre (-87.3593, -30.7028) end of major axis (-86.4944, -30.7085) minor radius 0.136 (-86.4957, -30.7008) -> (-87.5033, -30.5678) ccw
  ellipse E225 centre (-87.3528, -29.7153) end of major axis (-86.4878, -29.721) minor radius 0.136 (-86.4928, -29.7063) -> (-87.9483, -29.6128) ccw
  ellipse E226 centre (-97.0015, 42.174) end of major axis (-96.9356, 42.9143) minor radius 0.1949 (-96.7965, 42.3957) -> (-97.2065, 41.9524) ccw
  line L261 (-97.2065, 39.9427) -> (-97.2065, 41.9524)
  line L262 (-96.7965, 40.3855) -> (-96.7965, 42.3957)
  ellipse E227 centre (-94.8672, 42.1745) end of major axis (-94.7241, 42.9286) minor radius 0.1955 (-94.6401, 42.3749) -> (-94.915, 42.7042) ccw
  line L263 (-97.3506, 20.4086) -> (-97.2665, 21.2127)
  line L264 (-94.8015, 40.8328) -> (-94.6401, 42.3749)
  ellipse E228 centre (-99.1359, 42.1745) end of major axis (-99.152, 42.9419) minor radius 0.1955 (-99.1101, 42.9252) -> (-99.3166, 41.9316) ccw
  line L265 (-99.2114, 40.9268) -> (-99.3166, 41.9316)
  line L266 (-96.6525, 20.4086) -> (-96.7366, 21.2127)
  ellipse E229 centre (-97.0015, 40.1641) end of major axis (-96.9354, 40.9011) minor radius 0.1948 (-96.7965, 40.3855) -> (-97.2065, 39.9427) ccw
  line L267 (-97.2065, 23.4075) -> (-97.2065, 39.9427)
  line L268 (-96.7965, 23.4075) -> (-96.7965, 40.3855)
  ellipse E230 centre (-94.8361, 40.164) end of major axis (-94.6838, 40.9163) minor radius 0.1955 (-94.6066, 40.3616) -> (-94.9051, 40.6287) ccw
  line L269 (-98.1701, 13.3945) -> (-97.3506, 20.4087)
  line L270 (-96.7846, 21.7196) -> (-94.6066, 40.3616)
  line L271 (-97.2065, 13.3927) -> (-97.2065, 19.8971)
  line L272 (-96.7965, 13.3927) -> (-96.7965, 19.8971)
  ellipse E231 centre (-99.167, 40.164) end of major axis (-99.1924, 40.9311) minor radius 0.1955 (-99.127, 40.8909) -> (-99.3448, 39.9189) ccw
  line L273 (-97.2184, 21.7196) -> (-99.3448, 39.9189)
  line L274 (-95.833, 13.3945) -> (-96.6525, 20.4087)
  ellipse E232 centre (-97.0015, 44.2021) end of major axis (-96.9377, 44.967) minor radius 0.1955 (-96.7965, 44.425) -> (-97.2065, 43.9793) ccw
  line L275 (-97.2065, 43.9582) -> (-97.2065, 43.9793)
  line L276 (-96.7965, 44.402) -> (-96.7965, 44.425)
  ellipse E233 centre (-97.0015, 44.1801) end of major axis (-96.9358, 44.9231) minor radius 0.1949 (-96.7965, 44.402) -> (-97.2065, 43.9582) ccw
  line L277 (-97.2065, 41.9524) -> (-97.2065, 43.9582)
  line L278 (-96.7965, 42.3957) -> (-96.7965, 44.402)
  ellipse E234 centre (-94.8835, 44.1809) end of major axis (-94.7477, 44.9364) minor radius 0.1955 (-94.6584, 44.3835) -> (-95.1086, 43.9783) ccw
  ellipse E235 centre (-97.8026, 13.3841) end of major axis (-97.5985, 13.3647) minor radius 0 (-97.5985, 13.3647) -> (-97.8444, 13.388) ccw
  line L279 (-97.2666, 21.2118) -> (-97.2184, 21.7197)
  line L280 (-96.7965, 26.1706) -> (-95.1086, 43.9783)
  line L281 (-97.5985, 13.3647) -> (-97.2065, 17.5001)
  line L282 (-94.7995, 42.8944) -> (-94.6584, 44.3835)
  ellipse E236 centre (-99.1196, 44.1809) end of major axis (-99.1282, 44.9485) minor radius 0.1955 (-98.9365, 44.4221) -> (-99.3026, 43.9398) ccw
  ellipse E237 centre (-96.2005, 13.3841) end of major axis (-96.4046, 13.3647) minor radius 0 (-96.1587, 13.388) -> (-96.4046, 13.3647) ccw
  line L283 (-96.4046, 13.3647) -> (-96.7965, 17.5001)
  line L284 (-99.2051, 42.9111) -> (-99.3026, 43.9398)
  line L285 (-96.7365, 21.2118) -> (-96.7847, 21.7197)
  line L286 (-97.2065, 26.1706) -> (-98.9365, 44.4221)
  line L287 (-106.0535, -29.3516) -> (-106.0278, -29.3367)
  line L288 (-106.112, -29.2317) -> (-106.1048, -29.2332)
  line L289 (-106.1383, -29.247) -> (-106.112, -29.2317)
  line L290 (-106.112, -29.2317) -> (-106.1089, -29.2018)
  line L291 (-107.7169, -29.1991) -> (-107.6996, -29.1999)
  line L292 (-107.6996, -29.1999) -> (-107.6522, -29.1801)
  line L293 (-107.5487, -29.1368) -> (-107.5155, -29.1229)
  line L294 (-107.3444, -29.0513) -> (-107.3202, -29.0412)
  line L295 (-107.5135, -29.0321) -> (-107.3202, -29.0412)
  line L296 (-107.5951, -29.0663) -> (-107.5135, -29.0321)
  line L297 (-107.3202, -29.0412) -> (-107.3203, -29.0399)
  line L298 (-107.5135, -29.0321) -> (-107.5149, -28.9756)
  line L299 (-107.5613, -27.1318) -> (-107.5613, -27.1315)
  line L300 (-107.6141, -25.0378) -> (-107.6147, -25.013)
  line L301 (-106.9497, -28.9802) -> (-106.9868, -28.9958)
  line L302 (-106.95, -28.9672) -> (-106.9497, -28.9802)
  line L303 (-106.9497, -28.9802) -> (-106.8322, -28.9857)
  line L304 (-106.6823, -28.9927) -> (-106.1982, -29.0153)
  line L305 (-87.7662, -29.0626) -> (-87.7393, -29.0604)
  line L306 (-87.4958, -29.0399) -> (-87.487, -29.0392)
  line L307 (-87.2319, -28.9759) -> (-87.2065, -28.9831)
  line L308 (-87.2912, -28.9809) -> (-87.2319, -28.9759)
  line L309 (-87.2319, -28.9759) -> (-87.2314, -28.9572)
  line L310 (-86.8113, -28.9331) -> (-86.8137, -29.0266)
  line L311 (-86.6375, -29.0118) -> (-86.8137, -29.0266)
  line L312 (-86.5362, -24.9912) -> (-86.5366, -25.0094)
  line L313 (-86.5896, -27.1111) -> (-86.5901, -27.1323)
  line L314 (-86.6358, -28.9446) -> (-86.6375, -29.0118)
  line L315 (-86.8137, -29.0266) -> (-86.6898, -29.0616)
  line L316 (-86.4074, -29.1416) -> (-86.3944, -29.1453)
  line L317 (-86.6375, -29.0118) -> (-86.479, -29.0566)
  line L318 (-86.329, -29.2316) -> (-86.3474, -29.2264)
  line L319 (-87.8708, -29.0855) -> (-87.8579, -29.0878)
  line L320 (-107.6516, -29.3057) -> (-107.8772, -29.2981)
  line L321 (-107.9651, -29.3365) -> (-107.8772, -29.2981)
  line L322 (-107.6495, -29.3472) -> (-107.9651, -29.3365)
  line L323 (-107.9651, -29.3365) -> (-107.9675, -29.2896)
  line L324 (-108.1749, -29.2447) -> (-107.9845, -29.2511)
  line L325 (-108.1777, -29.1897) -> (-108.1749, -29.2447)
  line L326 (-107.9845, -29.2511) -> (-107.5782, -29.0736)
  line L327 (-107.7686, -29.0672) -> (-107.5782, -29.0736)
  line L328 (-108.1749, -29.2447) -> (-107.7686, -29.0672)
  line L329 (-107.5782, -29.0736) -> (-107.5785, -29.0672)
  line L330 (-107.7686, -29.0672) -> (-107.7691, -29.0577)
  line L331 (-107.401, -24.9983) -> (-107.3995, -25.0287)
  line L332 (-87.0813, -29.0499) -> (-87.0782, -29.0497)
  line L333 (-86.8628, -29.0374) -> (-86.8041, -29.034)
  line L334 (-86.9112, -28.9964) -> (-86.8041, -29.034)
  line L335 (-86.9669, -28.9996) -> (-86.9112, -28.9964)
  line L336 (-86.8041, -29.034) -> (-86.8038, -29.0293)
  line L337 (-86.9112, -28.9964) -> (-86.9083, -28.9386)
  line L338 (-86.816, -27.1133) -> (-86.8154, -27.1014)
  line L339 (-86.5027, -29.0584) -> (-86.5029, -29.0625)
  line L340 (-86.3226, -29.0521) -> (-86.5029, -29.0625)
  line L341 (-86.3216, -29.033) -> (-86.3226, -29.0521)
  line L342 (-86.5029, -29.0625) -> (-86.0082, -29.2359)
  line L343 (-85.8279, -29.2256) -> (-86.0082, -29.2359)
  line L344 (-86.3226, -29.0521) -> (-85.8279, -29.2256)
  line L345 (-85.8279, -29.2256) -> (-85.8252, -29.1728)
  line L346 (-85.9778, -29.3237) -> (-86.0849, -29.2861)
  line L347 (-85.9753, -29.2747) -> (-85.9778, -29.3237)
  line L348 (-86.0849, -29.2861) -> (-86.3512, -29.3014)
  line L349 (-85.9778, -29.3237) -> (-86.3534, -29.3453)
  line L350 (-107.1367, -29.0353) -> (-107.0698, -29.0137)
  line L351 (-107.2578, -29.0002) -> (-107.0698, -29.0137)
  line L352 (-107.3656, -29.035) -> (-107.2578, -29.0002)
  line L353 (-107.0698, -29.0137) -> (-107.0701, -28.9631)
  line L354 (-107.0823, -27.1105) -> (-107.0851, -26.6881)
  line L355 (-107.2578, -29.0002) -> (-107.2581, -28.9568)
  line L356 (-107.2703, -27.1017) -> (-107.2704, -27.0958)
  line L357 (-107.2842, -24.9984) -> (-107.2844, -24.9716)
  line L358 (-88.0027, -29.0555) -> (-87.2778, -28.995)
  line L359 (-87.382, -28.9657) -> (-87.2778, -28.995)
  line L360 (-87.658, -28.9887) -> (-87.382, -28.9657)
  line L361 (-87.2778, -28.995) -> (-87.2777, -28.9851)
  line L362 (-87.382, -28.9657) -> (-87.3818, -28.9435)
  line L363 (-87.3556, -24.968) -> (-87.3554, -24.937)
  line L364 (-104.4345, -10.8414) -> (-105.4298, -10.7374)
  line L365 (-108.2282, -9.9422) -> (-105.3777, -10.2401)
  ellipse E238 centre (-106.0751, -10.1676) end of major axis (-108.5616, -9.9074) minor radius 0.0002 (-108.2282, -9.9422) -> (-108.5616, -9.9074) ccw
  line L366 (-108.7591, -11.7954) -> (-108.5616, -9.9074)
  line L367 (-88.5733, -10.7374) -> (-89.5685, -10.8414)
  line L368 (-88.6253, -10.2401) -> (-85.7749, -9.9422)
  ellipse E239 centre (-87.928, -10.1676) end of major axis (-85.4415, -9.9074) minor radius 0.0002 (-85.4415, -9.9074) -> (-85.7749, -9.9422) ccw
  line L369 (-85.4415, -9.9074) -> (-85.244, -11.7954)
  ellipse E240 centre (-105.8011, -14.6579) end of major axis (-106.0494, -14.6288) minor radius 0
  ellipse E241 centre (-104.7327, -14.7827) end of major axis (-105.3256, -14.7135) minor radius 0 (-105.2747, -14.7194) -> (-105.2747, -14.7194) ccw
  ellipse E242 centre (-108.2217, -14.3753) end of major axis (-107.4312, -14.4676) minor radius 0 (-108.5712, -14.3344) -> (-108.5713, -14.3345) ccw
  line L370 (-105.2747, -14.7192) -> (-109.1148, -14.2709)
  ellipse E243 centre (-106.9645, -14.5222) end of major axis (-109.4476, -14.232) minor radius 0.0001 (-109.1075, -14.2717) -> (-109.4476, -14.232) ccw
  line L371 (-108.8247, -11.7877) -> (-105.9783, -12.1201)
  ellipse E244 centre (-106.6744, -12.039) end of major axis (-109.1575, -11.7489) minor radius 0.0001 (-108.8247, -11.7877) -> (-109.1575, -11.7489) ccw
  line L372 (-109.4476, -14.232) -> (-109.1575, -11.7489)
  ellipse E245 centre (-101.3027, -15.1836) end of major axis (-109.7453, -14.1972) minor radius 0.0004 (-109.3236, -14.2466) -> (-108.5714, -14.3345) ccw
  line L373 (-105.0427, -12.7327) -> (-106.0364, -12.6167)
  ellipse E246 centre (-88.2019, -14.6579) end of major axis (-88.4503, -14.6869) minor radius 0
  ellipse E247 centre (-89.2704, -14.7827) end of major axis (-88.6775, -14.7135) minor radius 0 (-88.7284, -14.7194) -> (-88.7284, -14.7194) ccw
  ellipse E248 centre (-92.7004, -15.1836) end of major axis (-84.2578, -14.1972) minor radius 0.0004 (-85.4316, -14.3345) -> (-84.6794, -14.2466) ccw
  ellipse E249 centre (-87.0385, -14.5222) end of major axis (-84.5554, -14.232) minor radius 0.0001 (-84.6794, -14.2466) -> (-84.8882, -14.2709) ccw
  line L374 (-84.8882, -14.2709) -> (-88.7284, -14.7192)
  line L375 (-88.0247, -12.1201) -> (-85.1784, -11.7877)
  ellipse E250 centre (-87.3287, -12.039) end of major axis (-84.8456, -11.7489) minor radius 0.0001 (-84.8456, -11.7489) -> (-85.1784, -11.7877) ccw